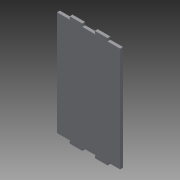
# Autodesk Inventor part: repisaa
Saved by Autodesk Inventor 2015 (Build 190159000, 159)
## iProperties
Created: 2016-01-26
Part Number: repisaa
Material: Generic
Document SubType Name: Modeling
Designer: iberopuebla
Density: 1 g/cm^3
Appearance: Default
Author: iberopuebla
Autodesk Inventor part; units mm, degrees
ref_plane "YZ Plane" through (0, 0, 0) normal (1, 0, 0) x (0, 1, 0)
ref_plane "XZ Plane" through (0, 0, 0) normal (0, 1, 0) x (-1, 0, 0)
ref_plane "XY Plane" through (0, 0, 0) normal (0, 0, 1) x (1, 0, 0)
sketch "Sketch1" plane through (0, 0, 0) normal (0, 1, 0) x (-1, 0, 0)
  line L0 (400, 0) -> (400, -664)
  line L1 (0, -664) -> (0, 0)
  line L2 (320, 2.5) -> (320, 18)
  line L3 (80, 2.5) -> (80, 18)
  line L4 (320, 18) -> (240, 18)
  line L5 (160, 18) -> (80, 18)
  line L6 (322.5, 0) -> (400, 0)
  line L7 (0, 0) -> (77.5, 0)
  line L8 (162.5, 0) -> (237.5, 0)
  arc A0 (320, 2.5) -> (322.5, 0) centre (320, 0) ccw
  arc A1 (237.5, 0) -> (240, 2.5) centre (240, 0) ccw
  arc A2 (160, 2.5) -> (162.5, 0) centre (160, 0) ccw
  arc A3 (77.5, 0) -> (80, 2.5) centre (80, 0) ccw
  line L9 (240, 18) -> (240, 2.5)
  line L10 (160, 18) -> (160, 2.5)
  line L11 (320, -666.5) -> (320, -682)
  line L12 (80, -666.5) -> (80, -682)
  line L13 (320, -682) -> (240, -682)
  line L14 (160, -682) -> (80, -682)
  line L15 (322.5, -664) -> (400, -664)
  line L16 (0, -664) -> (77.5, -664)
  line L17 (162.5, -664) -> (237.5, -664)
  arc A4 (322.5, -664) -> (320, -666.5) centre (320, -664) ccw
  arc A5 (240, -666.5) -> (237.5, -664) centre (240, -664) ccw
  arc A6 (162.5, -664) -> (160, -666.5) centre (160, -664) ccw
  arc A7 (80, -666.5) -> (77.5, -664) centre (80, -664) ccw
  line L18 (240, -682) -> (240, -666.5)
  line L19 (160, -682) -> (160, -666.5)
  dimension "d4" = 80
  dimension "d13" = 18
  dimension "d20" = 5
  dimension "d21" = 5
  dimension "d22" = 5
  dimension "d23" = 5
  dimension "d28" = 80
  dimension "d29" = 18
  dimension "d30" = 80
  dimension "d31" = 18
  dimension "d33" = 80
  dimension "d34" = 18
  dimension "d36" = 18
  dimension "d37" = 664
  constraints: 40 end point, 16 point on circle, 11 horizontal, 8 centre point, 7 perpendicular, 7 vertical, 1 parallel, 1 vertical alignment, 22 other
  measures "d4" distance from line of L3 L1.end
  measures "d13" vertical distance of L1.end L3.end
  measures "d20" diameter of A0
  measures "d21" diameter of A1
  measures "d22" diameter of A2
  measures "d23" diameter of A3
  measures "d28" distance of L0.start A0.centre
  measures "d29" distance of L2.end A0.centre
  measures "d30" distance of L2.end L4.end
  measures "d31" distance of L4.end A1.centre
  measures "d33" distance of A2.centre A1.centre
  measures "d34" distance from line of A2.centre L5
  measures "d36" distance from line of L0.start L4
  measures "d37" distance of L0.start L0.end
extrude "Extrusion1" add sketch "Sketch1" along normal blind 18
body "Solid1"
